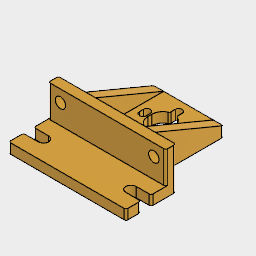
Z_Nut_Bracket_1.0_F01 (Autodesk Fusion 360 design; units mm, degrees)
Autodesk Fusion 360 part; units mm, degrees
sketch "スケッチ1" plane through (0, 0, 0) normal (0, 0, 1) x (1, 0, 0)
  line L0 (-17.5, 0) -> (-17.5, 36)
  line L1 (-17.5, 36) -> (17.5, 36)
  line L2 (17.5, 36) -> (17.5, 0)
  line L3 (-29.5, 0) -> (29.5, 0)
  line L4 (29.5, 0) -> (29.5, -25)
  line L5 (29.5, -25) -> (-29.5, -25)
  line L6 (-29.5, -25) -> (-29.5, 0)
  line L7 (-29.5, -5) -> (29.5, -5)
  line L8 (-12.5, 0) -> (-12.5, 36)
  line L9 (12.5, 0) -> (12.5, 36)
  circle A0 centre (22, -15) radius 2.6
  circle A1 centre (-22, -15) radius 2.6
  line L10 (29.5, -12.4) -> (22, -12.4)
  line L11 (29.5, -17.6) -> (22, -17.6)
  line L12 (-29.5, -12.4) -> (-22, -12.4)
  line L13 (-29.5, -17.6) -> (-22, -17.6)
  circle A2 centre (0, 23) radius 5.5
  circle A3 centre (0, 21) radius 5.5
  circle A4 centre (0, 31) radius 1.75
  circle A5 centre (0, 13) radius 1.75
  line L14 (0, 36) -> (0, 0) construction
  line L15 (1.75, 31) -> (1.75, 28.2142)
  line L16 (-1.75, 31) -> (-1.75, 28.2142)
  line L17 (1.75, 13) -> (1.75, 15.7858)
  line L18 (-1.75, 13) -> (-1.75, 15.7858)
  line L19 (5.5, 23) -> (5.5, 21)
  line L20 (-8, 23) -> (-8, 21)
  circle A6 centre (-8, 23) radius 1.75
  circle A7 centre (-8, 21) radius 1.75
  line L21 (-6.25, 21) -> (-6.25, 23)
  line L22 (-9.75, 21) -> (-9.75, 23)
  circle A8 centre (8, 23) radius 1.75
  line L23 (6.25, 21) -> (6.25, 23)
  circle A9 centre (8, 21) radius 1.75
  line L24 (9.75, 21) -> (9.75, 23)
  line L25 (-5.5, 23) -> (-5.5, 21)
  dimension "d1" = 36
  dimension "d2" = 25
  dimension "d3" = 5
  dimension "d4" = 35
  dimension "d5" = 59
  dimension "d6" = 17.5
  dimension "d7" = 5
  dimension "d8" = 5
  dimension "d9" = 5.2
  dimension "d10" = 5.2
  dimension "d11" = 7.5
  dimension "d12" = 7.5
  dimension "d13" = 10
  dimension "d14" = 10
  dimension "d15" = 11
  dimension "d16" = 11
  dimension "d17" = 3.5
  dimension "d18" = 3.5
  dimension "d19" = 5
  dimension "d20" = 18
  dimension "d21" = 2
  dimension "d22" = 8
  dimension "d23" = 2
  dimension "d24" = 3.5
  dimension "d25" = 3.5
  dimension "d26" = 8
  dimension "d27" = 8
  measures "d1" distance of L1.end L2.end
  measures "d2" distance of L3.end L4.end
  measures "d3" distance of L3 L7
  measures "d4" distance of L0 L2
  measures "d5" distance of L4.end L5.end
  measures "d6" distance of L14.end L0
  measures "d7" distance of L0 L8
  measures "d8" distance of L2 L9
  measures "d9" diameter of A0
  measures "d10" diameter of A1
  measures "d11" distance of L4 A0.centre
  measures "d12" distance of L6 A1.centre
  measures "d13" distance of L5 A0.centre
  measures "d14" distance of L5 A1.centre
  measures "d15" diameter of A2
  measures "d16" diameter of A3
  measures "d17" diameter of A4
  measures "d18" diameter of A5
  measures "d19" distance of L1 A4.centre
  measures "d20" distance of A4.centre A5.centre
  measures "d21" distance of A2.centre A3.centre
  measures "d22" distance of A2.centre A4.centre
  measures "d23" distance of L20.start L20.end
  measures "d24" diameter of A6
  measures "d25" diameter of A7
  measures "d26" distance of A2.centre L20.start
  measures "d27" distance of A4.centre L20.start
extrude "押し出し1" add sketch "スケッチ1" along normal blind 5 contours L3 L4 L6 L7 | L1 L3 L8 L9 | L4 L5 L6 L7 A0 A1 L10 L11 L12 L13
extrude "押し出し2" add sketch "スケッチ1" along normal blind 21 contours L3 L4 L6 L7
extrude "押し出し3" add sketch "スケッチ1" along normal blind 20 contours L0 L1 L3 L8 | L1 L2 L3 L9
chamfer "面取り1" distance 36 distance2 15 2 edges at (-15, 36, 20) (15, 36, 20) measured on face at (-15.8333, 24, 20) measured on face at (14.1667, 12, 20)
hole "穴1" at (23.5, -5, 15) direction (0, 1, 0) diameter 5.2 depth 6 tip angle 118
hole "穴2" at (-23.5, -5, 15) direction (0, 1, 0) diameter 5.2 depth 6 tip angle 118
fillet "フィレット1" radius 1 12 edges at (29.5, -25, 2.5) (29.5, -17.6, 2.5) (29.5, -12.4, 2.5) (29.5, -5, 13) (29.5, 0, 10.5) (17.5, 36, 2.5) (-17.5, 36, 2.5) (-29.5, 0, 10.5) (-29.5, -5, 13) (-29.5, -25, 2.5) (-29.5, -17.6, 2.5) (-29.5, -12.4, 2.5)
fillet "フィレット2" radius 1 4 edges at (1.75, 28.2142, 2.5) (1.75, 15.7858, 2.5) (-1.75, 15.7858, 2.5) (-1.75, 28.2142, 2.5)
equation "d6 = d4 / 2"
